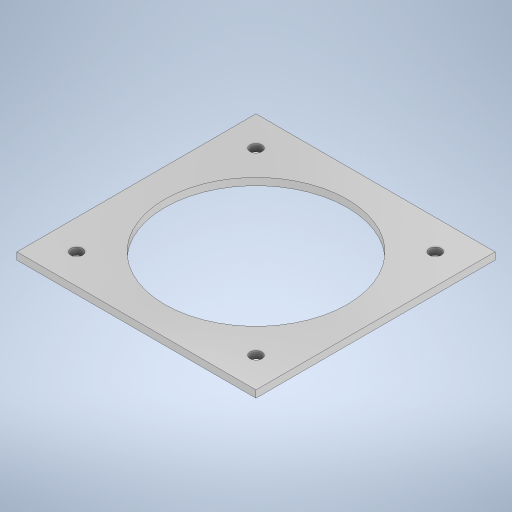
# Autodesk Inventor part: Plant Panel
Saved by Autodesk Inventor 2024 (Build 280153000, 153)
## iProperties
Created: 2023-07-19
Part Number: Plant Panel
Material: Aluminum 6061
Document SubType Name: Modeling
Designer: javie
Density: 2.7 g/cm^3
Appearance: Aluminum - Polished
Author: javie
Autodesk Inventor part; units mm, degrees
ref_plane "YZ Plane" through (0, 0, 0) normal (1, 0, 0) x (0, 1, 0)
ref_plane "XZ Plane" through (0, 0, 0) normal (0, 1, 0) x (-1, 0, 0)
ref_plane "XY Plane" through (0, 0, 0) normal (0, 0, 1) x (1, 0, 0)
sketch "Sketch1" plane through (0, 0, 0) normal (0, 1, 0) x (-1, 0, 0)
  line L0 (-50, 50) -> (50, 50)
  line L1 (50, 50) -> (50, -50)
  line L2 (50, -50) -> (-50, -50)
  line L3 (-50, -50) -> (-50, 50)
  line L4 (-50, 50) -> (50, -50) construction
  line L5 (50, 50) -> (-50, -50) construction
  point P0 (0, 0)
  dimension "d0" = 100
  dimension "d1" = 100
  constraints: 12 end point, 2 midpoint, 2 parallel, 1 horizontal, 1 perpendicular
  measures "d0" distance of L1.end L2.end
  measures "d1" distance of L0.end L1.end
extrude "Extrusion1" add sketch "Sketch1" along normal blind 3
sketch "Sketch2" plane through (0, 3, 0) normal (0, 1, 0) x (1, 0, 0)
  point P0 (0, 0)
  point P1 (0, 0)
  constraints: 1 coincident
hole "Hole1" at (0, 3, 0) direction (0, -1, 0) diameter 76.3 end through all
sketch "Sketch3" plane through (0, 3, 0) normal (0, 1, 0) x (1, 0, 0)
  line L0 (-50, -50) -> (50, -50) projected
  line L1 (-50, 50) -> (-50, -50) projected
  point P0 (0, 0)
  point P1 (-37.5, -37.5)
  point P2 (37.5, -37.5)
  point P3 (0, 0)
  point P4 (37.5, 37.5)
  point P5 (0, 0)
  point P6 (-37.5, 37.5)
  point P7 (0, 0)
  dimension "d18" = 12.5
  dimension "d19" = 12.5
  dimension "d22" = 360
  constraints: 2 coincident, 7 other
  measures "d18" distance from line of L0 point (-37.5, -37.5)
  measures "d19" distance from line of L1 point (-37.5, -37.5)
hole "Hole2" at (-37.5, 3, 37.5) at (-37.5, 3, -37.5) at (37.5, 3, -37.5) at (37.5, 3, 37.5) direction (0, -1, 0) diameter 5 end through all
body "Solid1"
